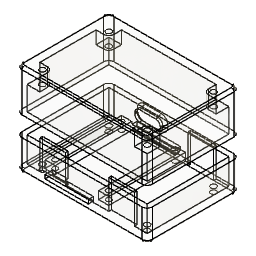
Enclosure (Autodesk Fusion 360 design; units mm, degrees)
Autodesk Fusion 360 part; units mm, degrees
sketch "Sketch1" plane through (0, 0, 0) normal (0, 0, 1) x (1, 0, 0) in component "Enclosure-Bottom"
  line L0 (0, 0) -> (45, 0) construction
  line L1 (45, 0) -> (45, 30) construction
  line L2 (45, 30) -> (0, 30) construction
  line L3 (0, 30) -> (0, 0) construction
  line L4 (-1, -1) -> (46, -1)
  line L5 (46, -1) -> (46, 31)
  line L6 (46, 31) -> (-1, 31)
  line L7 (-1, 31) -> (-1, -1)
  line L8 (-1, -3) -> (46, -3)
  line L9 (48, -1) -> (48, 31)
  line L10 (46, 33) -> (-1, 33)
  line L11 (-3, 31) -> (-3, -1)
  arc A0 (48, 31) -> (46, 33) centre (46, 31) ccw
  arc A1 (-1, 33) -> (-3, 31) centre (-1, 31) ccw
  arc A2 (-3, -1) -> (-1, -3) centre (-1, -1) ccw
  arc A3 (46, -3) -> (48, -1) centre (46, -1) ccw
  dimension "d1" = 45
  dimension "d2" = 30
  dimension "d5" = 1
  dimension "d9" = 2
  dimension "d23" = 3
  dimension "d25" = 3
  dimension "d26" = 3
  dimension "d27" = 3
  constraint horizontal L0
  constraint vertical L1
  constraint horizontal L2
  constraint vertical L3
  constraint coincident L0.start L3.end
  constraint parallel L0 L8
  constraint parallel L1 L9
  constraint parallel L2 L10
  constraint parallel L3 L11
  constraint tangent L9 A0
  constraint tangent L10 A0
  constraint tangent L10 A1
  constraint tangent L11 A1
  constraint equal A0 A1
  constraint tangent L11 A2
  constraint tangent L8 A2
  constraint equal A0 A2
  constraint tangent L8 A3
  constraint tangent L9 A3
  constraint equal A0 A3
  measures "d1" distance of L1.end L2.end
  measures "d2" distance of L0.end L1.end
  measures "d9" radius of A0
  measures "d23" distance of L2 L10
  measures "d25" distance of L0 L8
  measures "d26" distance of L3 L11
  measures "d27" distance of L1 L9
extrude "Extrude1" add sketch "Sketch1" against normal blind 2 contours L4 L5 L6 L7 | L8 L9 L10 L11 A0 A1 A2 A3 makes body 1 in component "Enclosure-Bottom"
extrude "Extrude2" add sketch "Sketch1" along normal blind 10 bodies 1 in component "Enclosure-Bottom"
ref_plane "WorkPlane1" through (22.5, 15, 32) normal (0, 0, 1) x (1, 0, 0)
sketch "Sketch1 (2)" plane through (22.5, 15, 32) normal (0, 0, 1) x (1, 0, 0) in component "Enclosure-Top"
  line L0 (-23.5, -16) -> (23.5, -16)
  line L1 (-23.5, 16) -> (-23.5, -16)
  line L2 (23.5, 16) -> (-23.5, 16)
  line L3 (23.5, -16) -> (23.5, 16)
  line L4 (-23.5, -18) -> (23.5, -18)
  arc A0 (23.5, -18) -> (25.5, -16) centre (23.5, -16) ccw
  line L5 (25.5, -16) -> (25.5, 16)
  line L6 (-25.5, 16) -> (-25.5, -16)
  arc A1 (-25.5, -16) -> (-23.5, -18) centre (-23.5, -16) ccw
  line L7 (23.5, 18) -> (-23.5, 18)
  arc A2 (-23.5, 18) -> (-25.5, 16) centre (-23.5, 16) ccw
  arc A3 (25.5, 16) -> (23.5, 18) centre (23.5, 16) ccw
extrude "Extrude1'" add sketch "Sketch1 (2)" against normal blind 14.2857 separate body makes body 2 in component "Enclosure-Top"
extrude "Extrude2'" add sketch "Sketch1 (2)" along normal blind 2 contours L0 L1 L2 L3 | L4 A0 L5 L6 A1 L7 A2 A3 bodies 2 in component "Enclosure-Top"
fillet "Fillet1" radius 1 8 edges at (48, 15, 34) (47.4142, 32.4142, 34) (22.5, 33, 34) (-2.4142, 32.4142, 34) (-3, 15, 34) (-2.4142, -2.4142, 34) (22.5, -3, 34) (47.4142, -2.4142, 34) on bodies 2 in component "Enclosure-Top"
fillet "Fillet1'" radius 1 8 edges at (-3, 15, -2) (-2.4142, 32.4142, -2) (22.5, 33, -2) (47.4142, 32.4142, -2) (48, 15, -2) (47.4142, -2.4142, -2) (22.5, -3, -2) (-2.4142, -2.4142, -2) on bodies 1 in component "Enclosure-Bottom"
sketch "Sketch2" plane through (0, 0, 32) normal (0, 0, -1) x (1, 0, 0) in component "Enclosure-Top"
  line L0 (46, 1) -> (-1, 1)
  line L1 (-1, 1) -> (-1, -31)
  line L2 (-1, -31) -> (46, -31)
  line L3 (46, -31) -> (46, 1)
  line L4 (46, -2) -> (-1, -2) construction
  line L5 (2, 1) -> (2, -31) construction
  line L6 (-1, 1) -> (46, 1)
  line L7 (-1, -31) -> (-1, 1)
  line L8 (46, 1) -> (46, -31)
  line L9 (46, -31) -> (-1, -31)
  line L10 (22.5, 1) -> (22.5, -31) construction
  line L11 (46, -15) -> (-1, -15) construction
  line L12 (46, -28) -> (-1, -28) construction
  line L13 (43, 1) -> (43, -31) construction
  circle A0 centre (43, -2) radius 1.1
  line L14 (43, -4) -> (46, -4)
  line L15 (41, -2) -> (41, 1)
  arc A1 (41, -2) -> (43, -4) centre (43, -2) ccw
  circle A2 centre (2, -2) radius 1.1
  line L16 (4, -2) -> (4, 1)
  arc A3 (2, -4) -> (4, -2) centre (2, -2) ccw
  line L17 (2, -4) -> (-1, -4)
  circle A4 centre (2, -28) radius 1.1
  line L18 (4, -28) -> (4, -31)
  arc A5 (4, -28) -> (2, -26) centre (2, -28) ccw
  line L19 (2, -26) -> (-1, -26)
  line L20 (43, -26) -> (46, -26)
  circle A6 centre (43, -28) radius 1.1
  arc A7 (43, -26) -> (41, -28) centre (43, -28) ccw
  line L21 (41, -28) -> (41, -31)
  dimension "d28" = 3
  dimension "d29" = 3
  dimension "d30" = 2.2
  dimension "d31" = 4
  constraint coincident L3 L4.start
  constraint coincident L1 L4.end
  constraint perpendicular L1 L4
  constraint coincident L0 L5.start
  constraint coincident L2 L5.end
  constraint perpendicular L2 L5
  constraint midpoint L6 L10.start
  constraint midpoint L9 L10.end
  constraint midpoint L8 L11.start
  constraint midpoint L7 L11.end
  constraint symmetric L4.start L11 L12.start
  constraint symmetric L4.end L11 L12.end
  constraint symmetric L5.start L10 L13.start
  constraint symmetric L5.end L10 L13.end
  constraint coincident L13 A0.centre
  constraint coincident L4 A0.centre
  constraint concentric A0 A1
  constraint coincident L13 L14.start
  constraint coincident L8 L14.end
  constraint tangent L14 A1
  constraint coincident L4 L15.start
  constraint coincident L6 L15.end
  constraint tangent L15 A1
  constraint symmetric L10 A0 A2
  constraint symmetric L10 L14.start A3.start
  constraint symmetric L10 L14.end L17.end
  constraint symmetric L10 L15.start L16.start
  constraint symmetric L10 L15.end L16.end
  constraint symmetric L10 A1 A3
  constraint symmetric L11 A0 A6
  constraint symmetric L11 L14.start L20.start
  constraint symmetric L11 L14.end L20.end
  constraint symmetric L11 L15.start A7.end
  constraint symmetric L11 L15.end L21.end
  constraint symmetric L11 A1 A7
  constraint symmetric L11 A2 A4
  constraint symmetric L11 L16.start L18.start
  constraint symmetric L11 L16.end L18.end
  constraint symmetric L11 A3.start A5.end
  constraint symmetric L11 A3 A5
  constraint symmetric L11 L17.end L19.end
  measures "d28" distance of L0 L4
  measures "d29" distance of L5 L7
  measures "d30" diameter of A0
  measures "d31" diameter of A1
extrude "Extrude3" add sketch "Sketch2" along normal blind 5 contours L0 L3 L6 L8 L14 L15 A1 | L0 L1 L6 L7 L16 A3 L17 | L2 L3 L8 L9 L20 A7 L21 | L1 L2 L7 L9 L18 A5 L19 bodies 2 in component "Enclosure-Top"
sketch "Sketch2 (2)" plane through (0, 0, 0) normal (0, 0, 1) x (-1, 0, 0) in component "Enclosure-Bottom"
  line L0 (1, 1) -> (-46, 1)
  line L1 (-46, 1) -> (-46, -31)
  line L2 (-46, -31) -> (1, -31)
  line L3 (1, -31) -> (1, 1)
  line L4 (1, -31) -> (-46, -31)
  line L5 (-46, -31) -> (-46, 1)
  line L6 (1, 1) -> (1, -31)
  line L7 (-46, 1) -> (1, 1)
  line L8 (-22.5, -31) -> (-22.5, 1) construction
  line L9 (-46, -15) -> (1, -15) construction
  line L10 (-41, -31) -> (-41, -30)
  line L11 (-41, -30) -> (-31, -30)
  line L12 (-31, -30) -> (-31, -31)
  line L13 (-4, 1) -> (-4, 0)
  line L14 (-4, 0) -> (-14, 0)
  line L15 (-14, 0) -> (-14, 1)
  line L16 (-31, 0) -> (-31, 1)
  line L17 (-41, 0) -> (-31, 0)
  line L18 (-41, 1) -> (-41, 0)
  dimension "d44" = 10
  dimension "d45" = 1
  dimension "d46" = 5
  constraint midpoint L4 L8.start
  constraint midpoint L7 L8.end
  constraint midpoint L5 L9.start
  constraint midpoint L6 L9.end
  constraint vertical L10
  constraint horizontal L11
  constraint vertical L12
  constraint symmetric L9 L12.end L16.end
  constraint symmetric L9 L10.start L18.start
  constraint symmetric L9 L10.end L17.start
  constraint symmetric L9 L11.end L16.start
  measures "d44" distance of L12.end L10.start
  measures "d45" distance of L12.end L11.end
  measures "d46" distance of L5 L10
sketch "Sketch4" plane through (0, 0, -2) normal (0, 0, -1) x (1, 0, 0) in component "Enclosure-Bottom"
  line L0 (-2, 1) -> (-2, -31)
  arc A0 (-2, -31) -> (-1, -32) centre (-1, -31) ccw
  line L1 (-1, -32) -> (46, -32)
  arc A1 (46, -32) -> (47, -31) centre (46, -31) ccw
  line L2 (47, -31) -> (47, 1)
  arc A2 (47, 1) -> (46, 2) centre (46, 1) ccw
  line L3 (46, 2) -> (-1, 2)
  arc A3 (-1, 2) -> (-2, 1) centre (-1, 1) ccw
  circle A4 centre (43, -2) radius 1.1
  circle A5 centre (2, -2) radius 1.1
  circle A6 centre (2, -28) radius 1.1
  circle A7 centre (43, -28) radius 1.1
extrude "Extrude5" add sketch "Sketch2 (2)" along normal blind 11.4286 contours L0 L7 L13 L14 L15 | L2 L4 L10 L11 L12 | L0 L7 L16 L17 L18 bodies 1 in component "Enclosure-Bottom"
extrude "Extrude6" cut sketch "Sketch4" against normal blind 2 contours A4 | A5 | A6 | A7 bodies 1 in component "Enclosure-Bottom"
sketch "Sketch5" plane through (0, 0, 0) normal (0, 0, 1) x (-1, 0, 0) in component "Enclosure-Bottom"
  circle A0 centre (-43, -2) radius 1.1
  circle A1 centre (-2, -28) radius 1.1 construction
  circle A2 centre (-43, -28) radius 1.1
  circle A3 centre (-2, -2) radius 1.1
  line L0 (-4, 1) -> (-4, 0)
  line L1 (-4, 0) -> (-14, 0)
  line L2 (-14, 0) -> (-14, 1)
  line L3 (-14, 1) -> (-31, 1)
  line L4 (-31, 1) -> (-31, 0)
  line L5 (-31, 0) -> (-41, 0)
  line L6 (-41, 0) -> (-41, 1)
  line L7 (-41, 1) -> (-46, 1)
  line L8 (-46, 1) -> (-46, -31) construction
  line L9 (-46, -31) -> (-41, -31)
  line L10 (-41, -31) -> (-41, -30)
  line L11 (-41, -30) -> (-31, -30)
  line L12 (-31, -30) -> (-31, -31)
  line L13 (-31, -31) -> (1, -31)
  line L14 (1, -31) -> (1, 1) construction
  line L15 (1, 1) -> (-4, 1)
  line L16 (1, 1) -> (1, -31)
  line L17 (-46, -31) -> (-46, 1)
  circle A4 centre (-2, -28) radius 1.1
  line L18 (-4, -31) -> (-29, -31) construction
  line L19 (-29, -31) -> (-29, -1)
  line L20 (-29, -1) -> (-4, -1) construction
  line L21 (-4, -1) -> (-4, -31)
  line L22 (-6, -29) -> (-27, -29) construction
  line L23 (-27, -29) -> (-27, -3) construction
  line L24 (-27, -3) -> (-6, -3) construction
  line L25 (-6, -3) -> (-6, -29) construction
  circle A5 centre (-6, -29) radius 1
  circle A6 centre (-27, -29) radius 1
  circle A7 centre (-6, -3) radius 1
  circle A8 centre (-27, -3) radius 1
  line L26 (-25, -31) -> (-25, -1)
  line L27 (-8, -31) -> (-8, -1)
  line L28 (-4, -31) -> (-8, -31)
  line L29 (-4, -1) -> (-8, -1)
  line L30 (-29, -31) -> (-25, -31)
  line L31 (-29, -1) -> (-25, -1)
  line L32 (-41, -31) -> (-46, -31)
  line L33 (-4, 1) -> (1, 1)
  line L34 (-31, 1) -> (-14, 1)
  line L35 (1, -31) -> (-31, -31)
  line L36 (-46, 1) -> (-41, 1)
  dimension "d52" = 25
  dimension "d53" = 30
  dimension "d54" = 5
  dimension "d55" = 21
  dimension "d56" = 26
  dimension "d57" = 2
  dimension "d58" = 2
  dimension "d59" = 2
  dimension "d60" = 2
  dimension "d61" = 2
  dimension "d62" = 2
  dimension "d63" = 2
  dimension "d64" = 2
  constraint horizontal L18
  constraint vertical L19
  constraint horizontal L20
  constraint vertical L21
  constraint coincident L13.end L18
  constraint horizontal L22
  constraint vertical L23
  constraint horizontal L24
  constraint vertical L25
  constraint coincident L22.start L25.end
  constraint coincident L22.end L23.start
  constraint coincident L24.end L25.start
  constraint coincident L23.end L24.start
  constraint coincident L18 L26.start
  constraint coincident L20 L26.end
  constraint perpendicular L20 L26
  constraint coincident L18 L27.start
  constraint coincident L20 L27.end
  constraint perpendicular L20 L27
  measures "d52" distance of L18.start L18.end
  measures "d53" distance of L18.start L20.end
  measures "d54" distance of L14 L21
  measures "d55" distance of L22.start L22.end
  measures "d56" distance of L22.start L24.end
  measures "d57" distance of L21 L25
  measures "d58" distance of L20 L24
  measures "d59" diameter of A5
  measures "d60" diameter of A6
  measures "d61" diameter of A7
  measures "d62" diameter of A8
  measures "d63" distance of L23 L26
  measures "d64" distance of L25 L27
extrude "Extrude7" add sketch "Sketch5" along normal blind 3 contours L13 L21 L27 L28 L29 L35 | L13 L19 L26 L30 L31 L35 bodies 1 in component "Enclosure-Bottom"
sketch "Sketch6" plane through (0, 33, 0) normal (0, 1, 0) x (-1, 0, 0) in component "Enclosure-Bottom"
  line L0 (-46, -1) -> (1, -1)
  line L1 (1, -1) -> (1, 10)
  line L2 (1, 10) -> (-46, 10)
  line L3 (-46, 10) -> (-46, -1)
  line L4 (-14.6059, 4.3) -> (-10.9659, 4.3)
  arc A0 (-10.9659, 4.3) -> (-9.1859, 6.08) centre (-10.9659, 6.08) ccw
  line L5 (-9.1859, 6.08) -> (-9.1859, 6.68)
  arc A1 (-9.1859, 6.68) -> (-10.9659, 8.46) centre (-10.9659, 6.68) ccw
  line L6 (-10.9659, 8.46) -> (-17.3459, 8.46)
  arc A2 (-17.3459, 8.46) -> (-19.1259, 6.68) centre (-17.3459, 6.68) ccw
  line L7 (-19.1259, 6.68) -> (-19.1259, 6.08)
  arc A3 (-19.1259, 6.08) -> (-17.3459, 4.3) centre (-17.3459, 6.08) ccw
  line L8 (-17.3459, 4.3) -> (-14.6559, 4.3)
  line L9 (-14.6559, 4.3) -> (-14.6059, 4.3)
  constraint tangent L6 A2
  constraint tangent A1 L6
  constraint tangent L4 A0
  constraint tangent A0 L5
  constraint tangent L7 A3
  constraint tangent L5 A1
  constraint tangent A2 L7
  constraint tangent A3 L8
  constraint parallel L4 L9
extrude "Extrude8" cut sketch "Sketch6" against normal up to surface (2 mm away) contours L4 A0 L5 A1 L6 A2 L7 A3 L8 L9 bodies 1 in component "Enclosure-Bottom"
chamfer "Chamfer2" distance 1 angle 45 8 edges at (18.6046, 33, 7.9387) (14.1559, 33, 8.46) (9.7073, 33, 7.9387) (9.1859, 33, 6.38) (9.7073, 33, 4.8213) (14.1559, 33, 4.3) (18.6046, 33, 4.8213) (19.1259, 33, 6.38) on bodies 1 in component "Enclosure-Bottom"
sketch "Sketch7" plane through (0, 33, 0) normal (0, 1, 0) x (-1, 0, 0) in component "Enclosure-Bottom"
  line L0 (-46, -1) -> (1, -1)
  line L1 (1, -1) -> (1, 10)
  line L2 (1, 10) -> (-46, 10)
  line L3 (-46, 10) -> (-46, -1)
  arc A0 (-17.3459, 9.46) -> (-20.1259, 6.68) centre (-17.3459, 6.68) ccw
  line L4 (-17.3459, 9.46) -> (-10.9659, 9.46)
  arc A1 (-8.1859, 6.68) -> (-10.9659, 9.46) centre (-10.9659, 6.68) ccw
  line L5 (-8.1859, 6.68) -> (-8.1859, 6.08)
  arc A2 (-10.9659, 3.3) -> (-8.1859, 6.08) centre (-10.9659, 6.08) ccw
  line L6 (-10.9659, 3.3) -> (-17.3459, 3.3)
  arc A3 (-20.1259, 6.08) -> (-17.3459, 3.3) centre (-17.3459, 6.08) ccw
  line L7 (-20.1259, 6.08) -> (-20.1259, 6.68)
  line L8 (-25, 2) -> (-8, 2)
  line L9 (-8, 2) -> (-8, 0.5)
  line L10 (-8, 0.5) -> (-25, 0.5)
  line L11 (-25, 0.5) -> (-25, 2)
  dimension "d71" = 1.5
  constraint horizontal L8
  constraint vertical L9
  constraint horizontal L10
  constraint vertical L11
  measures "d71" distance of L8.start L10.end
extrude "Extrude9" cut sketch "Sketch7" against normal up to surface (36 mm away) contours L8 L9 L10 L11 bodies 1 in component "Enclosure-Bottom"
component "Enclosure-Bottom" placed x (1, 0, 0) y (0, 1, 0) z (0, 0, 1) at (0, 0, 0)
component "Enclosure-Top" placed x (1, 0, 0) y (0, 1, 0) z (0, 0, 1) at (0, 0, 0)
equation "d1 = length"
equation "d2 = width"
equation "wall_thickness = 2 mm"
equation "margin = 1 mm"
equation "d5 = margin"
equation "fillet_radius = 2 mm"
equation "height = 20 mm"
equation "d9 = fillet_radius"
equation "d10 = -wall_thickness"
equation "d12 = height / 2"
equation "d14 = height + wall_thickness"
equation "d15 = -height / 1.4"
equation "d17 = wall_thickness"
equation "d20 = 0.5 * fillet_radius"
equation "d22 = 0.5 * fillet_radius"
equation "d23 = wall_thickness + margin"
equation "d25 = wall_thickness + margin"
equation "d26 = wall_thickness + margin"
equation "d27 = wall_thickness + margin"
equation "d28 = 2 mm + margin"
equation "d29 = 2 mm + margin"
equation "d32 = height / 4"
equation "length = 45 mm"
equation "width = 30 mm"
equation "d44 = wall_thickness * 5"
equation "d45 = wall_thickness / 2"
equation "d47 = height / 1.75"
equation "d49 = -1 * wall_thickness"
equation "d56 = 30 mm - 2 mm - 2 mm"
